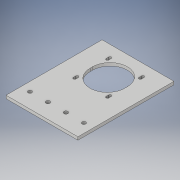
# Autodesk Inventor part: x motor mount (flattened)
Saved by Autodesk Inventor 2018.2 (Build 222227000, 227)
## iProperties
Created: 2018-01-30
Part Number: x motor mount (flattened)
Material: Generic
Document SubType Name: Modeling
Designer: torba
Density: 1 g/cm^3
Appearance: Default
Author: torba
Autodesk Inventor part; units mm, degrees
ref_plane "YZ Plane" through (0, 0, 0) normal (1, 0, 0) x (0, 1, 0)
ref_plane "XZ Plane" through (0, 0, 0) normal (0, 1, 0) x (-1, 0, 0)
ref_plane "XY Plane" through (0, 0, 0) normal (0, 0, 1) x (1, 0, 0)
sketch "Sketch1" plane through (0, 0, 0) normal (0, 1, 0) x (-1, 0, 0)
  line L0 (0, 0) -> (152.4, 0)
  line L1 (152.4, 0) -> (152.4, -203.6064)
  line L2 (152.4, -203.6064) -> (0, -203.6064)
  line L3 (0, -203.6064) -> (0, 0)
  line L4 (0, -203.6064) -> (152.4, -203.6064) construction
  line L5 (152.4, -203.6064) -> (152.4, -93.8561) construction
  line L6 (152.4, -93.8561) -> (0, -93.8561) construction
  line L7 (0, -203.6064) -> (0, -93.8561) construction
  arc A0 (108.1985, -179.0384) -> (113.7985, -179.0384) centre (110.9985, -179.0384) ccw
  line L8 (108.1985, -179.0384) -> (108.1985, -173.4384)
  arc A1 (113.7985, -173.4384) -> (108.1985, -173.4384) centre (110.9985, -173.4384) ccw
  line L9 (113.7985, -173.4384) -> (113.7985, -179.0384)
  arc A2 (38.6015, -179.0384) -> (44.2015, -179.0384) centre (41.4015, -179.0384) ccw
  line L10 (38.6015, -179.0384) -> (38.6015, -173.4384)
  arc A3 (44.2015, -173.4384) -> (38.6015, -173.4384) centre (41.4015, -173.4384) ccw
  line L11 (44.2015, -173.4384) -> (44.2015, -179.0384)
  arc A4 (38.6015, -109.4414) -> (44.2015, -109.4414) centre (41.4015, -109.4414) ccw
  line L12 (38.6015, -109.4414) -> (38.6015, -103.8414)
  arc A5 (44.2015, -103.8414) -> (38.6015, -103.8414) centre (41.4015, -103.8414) ccw
  line L13 (44.2015, -103.8414) -> (44.2015, -109.4414)
  arc A6 (108.1985, -109.4414) -> (113.7985, -109.4414) centre (110.9985, -109.4414) ccw
  line L14 (108.1985, -109.4414) -> (108.1985, -103.8414)
  arc A7 (113.7985, -103.8414) -> (108.1985, -103.8414) centre (110.9985, -103.8414) ccw
  line L15 (113.7985, -103.8414) -> (113.7985, -109.4414)
  arc A8 (39.4335, -144.2339) -> (112.9665, -144.2339) centre (76.2, -144.2339) ccw
  line L16 (39.4335, -144.2339) -> (39.4335, -138.6459)
  arc A9 (112.9665, -138.6459) -> (39.4335, -138.6459) centre (76.2, -138.6459) ccw
  line L17 (112.9665, -138.6459) -> (112.9665, -144.2339)
  circle A10 centre (57.15, -31.7483) radius 4.2164
  circle A11 centre (19.05, -31.7483) radius 3.9687
  circle A12 centre (133.35, -31.7483) radius 3.9687
  circle A13 centre (95.25, -31.7483) radius 4.2164
  line L18 (152.4, -53.4303) -> (152.4, 0) construction
  line L19 (0, 0) -> (152.4, 0) construction
  line L20 (0, -53.4303) -> (0, 0) construction
  line L21 (0, -53.4303) -> (152.4, -53.4303) construction
  dimension "d0" = 152.4
  dimension "d1" = 203.6064
  constraints: 44 end point, 20 point on circle, 14 centre point, 2 parallel, 1 horizontal, 1 perpendicular
  measures "d0" distance of L1.end L2.end
  measures "d1" distance of L0.end L1.end
extrude "Extrusion1" add sketch "Sketch1" along normal blind 6.35
body "Solid1"
